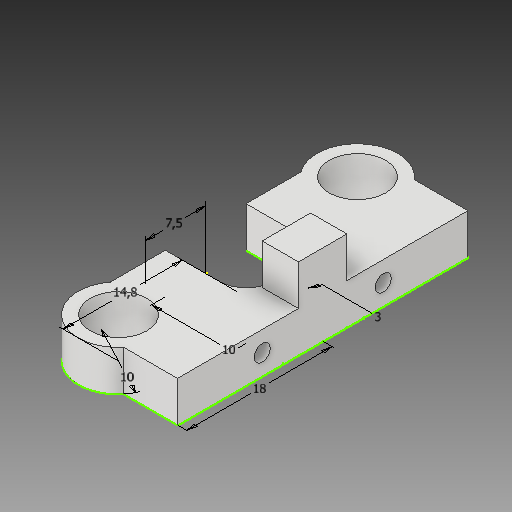
# Autodesk Inventor part: togh
Saved by Autodesk Inventor 2018 (Build 220112000, 112)
## iProperties
Created: 2017-05-26
Part Number: togh
Material: ABS Plastic
Document SubType Name: Modeling
Designer: Karol
Density: 1.06 g/cm^3
Appearance: Smooth - White
Author: Karol
Autodesk Inventor part; units mm, degrees
ref_plane "YZ Plane" through (0, 0, 0) normal (1, 0, 0) x (0, 1, 0)
ref_plane "XZ Plane" through (0, 0, 0) normal (0, 1, 0) x (-1, 0, 0)
ref_plane "XY Plane" through (0, 0, 0) normal (0, 0, 1) x (1, 0, 0)
sketch "Sketch1" plane through (0, 0, 0) normal (0, 1, 0) x (-1, 0, 0)
  line L0 (-3.25, 0) -> (-3.25, 1.7574)
  line L1 (-0.0074, 5) -> (6.75, 5)
  line L2 (-7.75, 0) -> (-7.75, 18)
  line L3 (-3.25, 0) -> (-3.25, -1.7574)
  line L4 (-0.0074, -5) -> (6.75, -5)
  line L5 (-7.75, 0) -> (-7.75, -17.9999)
  line L6 (6.75, -11.8) -> (6.75, -5)
  line L7 (-7.75, -17.9999) -> (-1.092, -17.9999)
  arc A0 (-1.092, -17.9999) -> (6.75, -11.8) centre (2.75, -14.8) ccw
  arc A1 (6.75, 11.8) -> (-1.0919, 18) centre (2.75, 14.8) ccw
  line L8 (6.75, 5) -> (6.75, 11.8)
  line L9 (-1.0919, 18) -> (-7.75, 18)
  line L10 (-2.1287, -4.1213) -> (-2.3713, -3.8787)
  line L11 (-2.1287, 4.1213) -> (-2.3713, 3.8787)
  arc A2 (-2.1287, -4.1213) -> (-0.0074, -5) centre (-0.0074, -2) ccw
  arc A3 (-3.25, -1.7574) -> (-2.3713, -3.8787) centre (-0.25, -1.7574) ccw
  arc A4 (-2.3713, 3.8787) -> (-3.25, 1.7574) centre (-0.25, 1.7574) ccw
  arc A5 (-0.0074, 5) -> (-2.1287, 4.1213) centre (-0.0074, 2) ccw
  line L12 (-0.0074, -5) -> (-3.25, -5)
  line L13 (-3.25, 5) -> (-0.0074, 5)
  line L14 (-3.25, -3) -> (-7.75, -3)
  line L15 (-3.25, 3) -> (-7.75, 3)
  line L16 (-3.25, -3) -> (-3.25, -1.7574)
  line L17 (-3.25, 3) -> (-3.25, 1.7574)
  line L18 (-3.25, -5) -> (-3.25, -3)
  line L19 (-3.25, 3) -> (-3.25, 5)
  point P0 (-1.25, 5)
  point P1 (-0.5666, 5)
  point P2 (-1.25, -5)
  point P3 (-0.5666, -5)
  point P4 (-7.75, -5)
  point P5 (-7.75, 5)
  point P6 (2.75, 0)
  dimension "d69" = 18
  dimension "d97" = 10
  dimension "d109" = 3
  dimension "d111" = 10
  dimension "d125" = 14.8
  constraints: 40 end point, 14 point on line, 12 point on circle, 11 tangent, 6 centre point, 4 collinear, 4 vertical, 3 equal radius, 3 horizontal, 2 coincident, 2 perpendicular, 1 parallel
  measures "d69" distance of L2.start L2.end
  measures "d97" diameter of A1
  measures "d109" radius of A2
  measures "d111" distance of L13.start L1.end
  measures "d125" distance of A1.centre point (2.75, 0)
extrude "Extrusion1" add sketch "Sketch1" along normal blind 5
hole "Hole5" at (-2.75, 0, 14.8) at (-2.75, 0, -14.8) direction (0, 1, 0) diameter 7 depth 8 tip angle 118
extrude "Wyciągnięcie proste11" add sketch "Sketch1" along normal blind 10 contours L3 L16 L14 L5 L2 L15 L17 L0
extrude "Wyciągnięcie proste12" cut sketch "Sketch1" along normal blind 1 contours L17 L19 L13 A5 L11 A4 | A3 L10 A2 L12 L18 L16
sketch "Szkic12" plane through (-6.75, 0, -11.8) normal (-1, 0, 0) x (0, 0, 1)
  point P0 (11.8, 0)
  point P1 (4.3, 2.5)
  point P2 (19.3, 2.5)
  dimension "d124" = 7.5
  measures "d124" horizontal distance of point (11.8, 0) point (19.3, 2.5)
hole "Otwór8" at (-6.75, 2.5, -7.5) at (-6.75, 2.5, 7.5) direction (1, 0, 0) diameter 2 end through all
body "Solid1"
